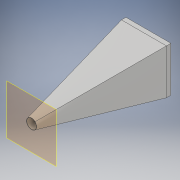
# Autodesk Inventor part: arrowadaptor
Saved by Autodesk Inventor 2018 (Build 220112000, 112)
## iProperties
Created: 2019-03-01
Part Number: arrowadaptor
Material: Generic
Document SubType Name: Modeling
Designer: F8PLTW
Density: 1 g/cm^3
Appearance: Default
Author: F8PLTW
Autodesk Inventor part; units mm, degrees
ref_plane "YZ Plane" through (0, 0, 0) normal (1, 0, 0) x (0, 1, 0)
ref_plane "XZ Plane" through (0, 0, 0) normal (0, 1, 0) x (-1, 0, 0)
ref_plane "XY Plane" through (0, 0, 0) normal (0, 0, 1) x (1, 0, 0)
sketch "Sketch1" plane through (0, 0, 0) normal (0, 0, 1) x (1, 0, 0)
  line L0 (-15.9951, 9.4971) -> (34.8049, 9.4971)
  line L1 (34.8049, 9.4971) -> (34.8049, -41.3029)
  line L2 (34.8049, -41.3029) -> (-15.9951, -41.3029)
  line L3 (-15.9951, -41.3029) -> (-15.9951, 9.4971)
  point P0 (0, 0)
  dimension "d0" = 50.8
  dimension "d1" = 50.8
  constraints: 8 end point, 2 parallel, 1 horizontal, 1 perpendicular
  measures "d0" distance of L1.end L2.end
  measures "d1" distance of L0.end L1.end
extrude "Extrusion1" add sketch "Sketch1" along normal blind 5.08
ref_plane "Work Plane1" through (0, 0, 132.08) normal (0, 0, 1) x (1, 0, 0)
sketch "Sketch2" plane through (0, 0, 5.08) normal (0, 0, 1) x (1, 0, 0)
  point P0 (0, 0)
sketch "Sketch3" plane through (0, 0, 132.08) normal (0, 0, 1) x (1, 0, 0)
  line L0 (34.8049, 9.4971) -> (-15.9951, 9.4971) projected
  line L1 (-15.9951, -41.3029) -> (34.8049, -41.3029) projected
  line L2 (-15.9951, 9.4971) -> (34.8049, -41.3029) construction
  line L3 (34.8049, 9.4971) -> (-15.9951, -41.3029) construction
  circle A0 centre (9.4049, -15.9029) radius 5.715
  point P0 (0, 0)
  dimension "d5" = 11.43
  constraints: 4 end point, 1 centre point, 1 midpoint
  measures "d5" diameter of A0
loft "Loft1" add profiles "Sketch3" section 1 edges at (9.4049, 9.4971, 5.08) (-15.9951, -15.9029, 5.08) (9.4049, -41.3029, 5.08) (34.8049, -15.9029, 5.08)
sketch "Sketch4" plane through (9.4049, -15.9029, 132.08) normal (0, 0, 1) x (1, 0, 0)
  circle A0 centre (0, 0) radius 5.3975
  point P0 (-9.4049, 15.9029)
  dimension "d11" = 10.795
  constraints: 1 centre point
  measures "d11" diameter of A0
extrude "Extrusion2" cut sketch "Sketch4" against normal blind 127
body "Solid1"
